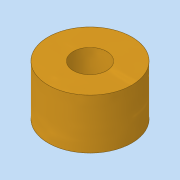
# Autodesk Inventor part: SleeveBearing2mm
Saved by Autodesk Inventor 2017 (Build 210142000, 142)
## iProperties
Created: 2017-03-04
Part Number: SleeveBearing2mm
Material: Brass, Soft Yellow, Welded
Document SubType Name: Modeling
Designer: techn
Density: 8.5 g/cm^3
Appearance: Weld - Brass
Author: techn
Autodesk Inventor part; units mm, degrees
ref_plane "YZ Plane" through (0, 0, 0) normal (1, 0, 0) x (0, 1, 0)
ref_plane "XZ Plane" through (0, 0, 0) normal (0, 1, 0) x (-1, 0, 0)
ref_plane "XY Plane" through (0, 0, 0) normal (0, 0, 1) x (1, 0, 0)
sketch "Sketch2" plane through (0, 0, 0) normal (0, 0, 1) x (1, 0, 0)
  line L0 (0, 0) -> (2.5, 0)
  line L1 (2.5, 0) -> (2.5, 3)
  line L2 (2.5, 3) -> (0, 3)
  line L3 (0, 3) -> (0, 0)
  line L4 (0, 3) -> (1, 3)
  line L5 (1, 3) -> (1, 0)
  line L6 (1, 0) -> (0, 0)
  line L7 (0, 0) -> (0, 3)
  dimension "d2" = 3
  dimension "d9" = 2.5
  dimension "d10" = 1
  constraints: 16 end point, 4 parallel, 2 horizontal, 2 perpendicular, 1 point on line
  measures "d2" distance of L1.end L0.end
  measures "d9" distance of L1.end L2.end
  measures "d10" distance of L5.end L6.end
revolve "Revolution2" add sketch "Sketch2" angle 360 about axis through (0, 3, 0) along (0, -1, 0) contours L5 L2 L1 L0
body "Solid2"
